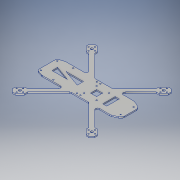
# Autodesk Inventor part: rama
Saved by Autodesk Inventor 2019 (Build 230136000, 136)
## iProperties
Created: 2020-11-11
Part Number: rama
Material: Aluminium 6061
Document SubType Name: Modeling
Designer: Karol
Density: 2.7 g/cm^3
Appearance: Aluminium — płaski
Mass: 121.616 g
Surface Area: 358.369 cm^2
Volume: 45.0429 cm^3
Author: Karol
Autodesk Inventor part; units mm, degrees
ref_plane "YZ Plane" through (0, 0, 0) normal (1, 0, 0) x (0, 1, 0)
ref_plane "XZ Plane" through (0, 0, 0) normal (0, 1, 0) x (-1, 0, 0)
ref_plane "XY Plane" through (0, 0, 0) normal (0, 0, 1) x (1, 0, 0)
sketch "Szkic1" plane through (0, 0, 0) normal (0, 1, 0) x (-1, 0, 0)
  line L0 (-112.8767, 0) -> (86.1409, 0) construction
  circle A0 centre (0, 0) radius 125 construction
  line L1 (0, 0) -> (-129.3005, -129.3005) construction
  line L2 (0, 0) -> (182.8585, 0) construction
  line L3 (0, 0) -> (-129.3005, 129.3005) construction
  circle A1 centre (-88.3883, -88.3883) radius 63.5 construction
  circle A2 centre (-88.3883, 88.3883) radius 63.5 construction
  line L4 (-88.3883, -88.3883) -> (-106.6347, -70.142) construction
  line L5 (-88.3883, -88.3883) -> (-62.5841, -88.3883) construction
  line L6 (0, 0) -> (0, 184.1198) construction
  line L7 (0, 0) -> (129.3005, -129.3005) construction
  line L8 (0, 0) -> (129.3005, 129.3005) construction
  circle A3 centre (88.3883, -88.3883) radius 63.5 construction
  circle A4 centre (88.3883, 88.3883) radius 63.5 construction
  circle A5 centre (70, -24.5) radius 1.5
  circle A6 centre (12, -24.5) radius 1.5
  circle A7 centre (70, 24.5) radius 1.5
  circle A8 centre (12, 24.5) radius 1.5
  line L9 (8.5, -28) -> (100, -28) construction
  line L10 (100, -28) -> (100, 0.6779) construction
  line L11 (8.5, 0) -> (8.5, -28) construction
  circle A9 centre (3.5, -15.283) radius 1.5
  circle A10 centre (-27.066, -15.283) radius 1.5
  circle A11 centre (3.5, 15.283) radius 1.5
  circle A12 centre (-27.066, 15.283) radius 1.5
  line L12 (-19.8579, -29) -> (0.4594, -29)
  line L13 (-75.6604, -82.7315) -> (-23.3934, -30.4645)
  arc A13 (-19.8579, -29) -> (-23.3934, -30.4645) centre (-19.8579, -34) ccw
  line L14 (-19.8579, 29) -> (0.4594, 29)
  arc A14 (-23.3934, 30.4645) -> (-19.8579, 29) centre (-19.8579, 34) ccw
  line L15 (48.1421, -29) -> (92.6893, -29)
  line L16 (19.8579, -29) -> (0.4594, -29)
  arc A15 (23.3934, -30.4645) -> (19.8579, -29) centre (19.8579, -34) ccw
  line L17 (19.8579, 29) -> (0.4594, 29)
  arc A16 (19.8579, 29) -> (23.3934, 30.4645) centre (19.8579, 34) ccw
  line L18 (-88.3883, -88.3883) -> (-88.3883, -65.5663) construction
  circle A17 centre (-80.3883, -88.3883) radius 1.5
  circle A18 centre (-88.3883, -80.3883) radius 1.5
  circle A19 centre (-88.3883, -88.3883) radius 3
  circle A20 centre (-88.3883, -96.3883) radius 1.5
  circle A21 centre (-96.3883, -88.3883) radius 1.5
  line L19 (-82.7315, -75.6604) -> (-89.8026, -75.6604)
  line L20 (-89.8026, -75.6604) -> (-101.1163, -86.9741)
  line L21 (-101.1163, -94.0452) -> (-101.1163, -86.9741)
  line L22 (-101.1163, -94.0452) -> (-97.5807, -97.5807)
  line L23 (-75.6604, -82.7315) -> (-75.6604, -89.8026)
  line L24 (-75.6604, -89.8026) -> (-86.9741, -101.1163)
  line L25 (-94.0452, -101.1163) -> (-86.9741, -101.1163)
  line L26 (-94.0452, -101.1163) -> (-97.5807, -97.5807)
  line L27 (-75.6604, 82.7315) -> (-23.3934, 30.4645)
  circle A22 centre (-80.3883, 88.3883) radius 1.5
  circle A23 centre (-88.3883, 80.3883) radius 1.5
  circle A24 centre (-88.3883, 88.3883) radius 3
  circle A25 centre (-88.3883, 96.3883) radius 1.5
  circle A26 centre (-96.3883, 88.3883) radius 1.5
  line L28 (-82.7315, 75.6604) -> (-89.8026, 75.6604)
  line L29 (-89.8026, 75.6604) -> (-101.1163, 86.9741)
  line L30 (-101.1163, 94.0452) -> (-101.1163, 86.9741)
  line L31 (-101.1163, 94.0452) -> (-97.5807, 97.5807)
  line L32 (-75.6604, 89.8026) -> (-86.9741, 101.1163)
  line L33 (-94.0452, 101.1163) -> (-86.9741, 101.1163)
  line L34 (-94.0452, 101.1163) -> (-97.5807, 97.5807)
  line L35 (-75.6604, 82.7315) -> (-75.6604, 89.8026)
  line L36 (88.3883, -88.3883) -> (106.6347, -70.142) construction
  line L37 (75.6604, -82.7315) -> (23.3934, -30.4645)
  line L38 (88.3883, -88.3883) -> (88.3883, -65.5663) construction
  circle A27 centre (80.3883, -88.3883) radius 1.5
  circle A28 centre (88.3883, -80.3883) radius 1.5
  circle A29 centre (88.3883, -88.3883) radius 3
  circle A30 centre (88.3883, -96.3883) radius 1.5
  circle A31 centre (96.3883, -88.3883) radius 1.5
  line L39 (82.7315, -75.6604) -> (89.8026, -75.6604)
  line L40 (89.8026, -75.6604) -> (101.1163, -86.9741)
  line L41 (101.1163, -94.0452) -> (101.1163, -86.9741)
  line L42 (101.1163, -94.0452) -> (97.5807, -97.5807)
  line L43 (75.6604, -89.8026) -> (86.9741, -101.1163)
  line L44 (94.0452, -101.1163) -> (86.9741, -101.1163)
  line L45 (94.0452, -101.1163) -> (97.5807, -97.5807)
  line L46 (75.6604, -82.7315) -> (75.6604, -89.8026)
  line L47 (75.6604, 82.7315) -> (23.3934, 30.4645)
  line L48 (75.6604, 89.8026) -> (86.9741, 101.1163)
  line L49 (94.0452, 101.1163) -> (86.9741, 101.1163)
  line L50 (82.7315, 75.6604) -> (89.8026, 75.6604)
  circle A32 centre (88.3883, 80.3883) radius 1.5
  circle A33 centre (80.3883, 88.3883) radius 1.5
  circle A34 centre (88.3883, 88.3883) radius 3
  line L51 (89.8026, 75.6604) -> (101.1163, 86.9741)
  circle A35 centre (96.3883, 88.3883) radius 1.5
  line L52 (101.1163, 94.0452) -> (101.1163, 86.9741)
  line L53 (101.1163, 94.0452) -> (97.5807, 97.5807)
  circle A36 centre (88.3883, 96.3883) radius 1.5
  line L54 (94.0452, 101.1163) -> (97.5807, 97.5807)
  line L55 (75.6604, 82.7315) -> (75.6604, 89.8026)
  line L56 (-196.7621, 0) -> (-196.7621, -23) construction
  line L57 (-196.7621, -23) -> (-302.8841, -23) construction
  line L58 (-302.8841, -23) -> (-302.8841, -70.142) construction
  line L59 (-302.8841, -70.142) -> (-413.5658, 0) construction
  line L60 (-196.7621, 0) -> (-196.7621, 23) construction
  line L61 (-196.7621, 23) -> (-302.8841, 23) construction
  line L62 (-302.8841, 23) -> (-302.8841, 70.142) construction
  line L63 (-302.8841, 70.142) -> (-413.5658, 0) construction
  line L64 (-82.7315, -75.6604) -> (-44.6066, -37.5355)
  arc A37 (-44.6066, -37.5355) -> (-48.1421, -29) centre (-48.1421, -34) ccw
  line L65 (82.7315, -75.6604) -> (44.6066, -37.5355)
  arc A38 (48.1421, -29) -> (44.6066, -37.5355) centre (48.1421, -34) ccw
  line L66 (94.2344, -28.7553) -> (106.5451, -24.7553)
  line L67 (110, -20) -> (110, 0)
  arc A39 (92.6893, -29) -> (94.2344, -28.7553) centre (92.6893, -24) ccw
  arc A40 (106.5451, -24.7553) -> (110, -20) centre (105, -20) ccw
  line L68 (-48.1421, -29) -> (-73.1421, -29)
  line L69 (-77.0275, -28.2143) -> (-88.8853, -23.2143)
  line L70 (-95, -14) -> (-95, 0)
  arc A41 (-77.0275, -28.2143) -> (-73.1421, -29) centre (-73.1421, -19) ccw
  arc A42 (-95, -14) -> (-88.8853, -23.2143) centre (-85, -14) ccw
  line L71 (48.1421, 29) -> (92.6893, 29)
  line L72 (-82.7315, 75.6604) -> (-44.6066, 37.5355)
  arc A43 (-48.1421, 29) -> (-44.6066, 37.5355) centre (-48.1421, 34) ccw
  arc A44 (44.6066, 37.5355) -> (48.1421, 29) centre (48.1421, 34) ccw
  line L73 (82.7315, 75.6604) -> (44.6066, 37.5355)
  line L74 (94.2344, 28.7553) -> (106.5451, 24.7553)
  line L75 (110, 20) -> (110, 0)
  arc A45 (110, 20) -> (106.5451, 24.7553) centre (105, 20) ccw
  line L76 (-48.1421, 29) -> (-73.1421, 29)
  line L77 (-77.0275, 28.2143) -> (-88.8853, 23.2143)
  line L78 (-95, 14) -> (-95, 0)
  arc A46 (-73.1421, 29) -> (-77.0275, 28.2143) centre (-73.1421, 19) ccw
  arc A47 (-88.8853, 23.2143) -> (-95, 14) centre (-85, 14) ccw
  arc A48 (94.2344, 28.7553) -> (92.6893, 29) centre (92.6893, 24) ccw
  point P0 (-96.6274, -86.0208)
  point P1 (-104.1875, -93.5809)
  point P2 (-99.7021, -99.7021)
  point P3 (-95, -29)
  point P4 (36.0711, -29)
  point P5 (93.4812, -29)
  point P6 (-85.5599, -88.3883)
  point P7 (-96.6274, 86.0208)
  point P8 (-85.5599, 88.3883)
  point P9 (96.6274, -86.0208)
  point P10 (104.1875, -93.5809)
  point P11 (99.7021, -99.7021)
  point P12 (85.5599, -88.3883)
  point P13 (96.6274, 86.0208)
  point P14 (85.5599, 88.3883)
  dimension "d0" = 250
  dimension "d1" = 135
  dimension "d3" = 127
  dimension "d4" = 127
  dimension "d10" = 135
  dimension "d12" = 3
  dimension "d13" = 24.5
  dimension "d14" = 58
  dimension "d15" = 70
  dimension "d16" = 3.5
  dimension "d17" = 28
  dimension "d19" = 30
  dimension "d20" = 3
  dimension "d22" = 5
  dimension "d23" = 15.283
  dimension "d32" = 5
  dimension "d37" = 30.566
  dimension "d64" = 3
  dimension "d65" = 8
  dimension "d66" = 8
  dimension "d67" = 6
  dimension "d70" = 10
  dimension "d73" = 5
  dimension "d74" = 13
  dimension "d75" = 5
  dimension "d76" = 5
  dimension "d77" = 110
  dimension "d78" = 20
  dimension "d79" = 29
  dimension "d80" = 18
  dimension "d81" = 91.5
  dimension "d82" = 10
  dimension "d83" = 95
  dimension "d84" = 14
  dimension "d85" = 25
  constraints: 158 end point, 103 symmetric about line, 49 centre point, 34 point on circle, 16 point on line, 13 tangent, 7 horizontal, 5 coincident, 5 equal radius, 5 perpendicular, 4 parallel, 4 vertical, 2 equal length, 1 collinear, 33 other
  measures "d0" diameter of A0
  measures "d1" angle of L1 L2
  measures "d3" diameter of A1
  measures "d4" diameter of A2
  measures "d10" angle of L5 L4
  measures "d12" diameter of A5
  measures "d13" vertical distance of point (0, 0) A5.centre
  measures "d14" distance of A5.centre A6.centre
  measures "d15" distance from line of L6 A5.centre
  measures "d16" distance from line of L11 A6.centre
  measures "d17" distance between parallel lines of L0 L9
  measures "d19" distance from line of A5.centre L10
  measures "d20" diameter of A9
  measures "d22" distance from line of A9.centre L11
  measures "d23" distance from line of L0 A9.centre
  measures "d32" radius of A13
  measures "d37" distance of A10.centre A9.centre
  measures "d64" diameter of A17
  measures "d65" distance from line of L5 A18.centre
  measures "d66" distance from line of L18 A17.centre
  measures "d67" diameter of A19
  measures "d70" distance between parallel lines of L1 L20
  measures "d73" distance from line of L1 L19.start
  measures "d74" distance from line of L22 A19.centre
  measures "d75" radius of A37
  measures "d76" radius of A39
  measures "d77" distance between parallel lines of L6 L67
  measures "d78" distance from line of L0 A40.centre
  measures "d79" distance between parallel lines of L0 L15
  measures "d80" angle of L66 L15
  measures "d81" distance between parallel lines of L10 L11
  measures "d82" radius of A41
  measures "d83" distance between parallel lines of L6 L70
  measures "d84" distance from line of L0 A42.centre
  measures "d85" horizontal distance of A37.centre A41.centre
extrude "Wyciągnięcie proste5" add sketch "Szkic1" along normal blind 3
sketch "Szkic2" plane through (0, 3, 0) normal (0, 1, 0) x (1, 0, 0)
  circle A0 centre (-88.3883, 88.3883) radius 3 projected
  circle A1 centre (-88.3883, -88.3883) radius 3 projected
  circle A2 centre (88.3883, -88.3883) radius 3 projected
  circle A3 centre (88.3883, 88.3883) radius 3 projected
  circle A4 centre (-88.3883, 96.3883) radius 1.5 projected
  circle A5 centre (-96.3883, 88.3883) radius 1.5 projected
  circle A6 centre (-88.3883, 80.3883) radius 1.5 projected
  circle A7 centre (-80.3883, 88.3883) radius 1.5 projected
  circle A8 centre (-96.3883, -88.3883) radius 1.5 projected
  circle A9 centre (-88.3883, -96.3883) radius 1.5 projected
  circle A10 centre (-88.3883, -80.3883) radius 1.5 projected
  circle A11 centre (-80.3883, -88.3883) radius 1.5 projected
  circle A12 centre (88.3883, -96.3883) radius 1.5 projected
  circle A13 centre (96.3883, -88.3883) radius 1.5 projected
  circle A14 centre (80.3883, -88.3883) radius 1.5 projected
  circle A15 centre (88.3883, -80.3883) radius 1.5 projected
  circle A16 centre (96.3883, 88.3883) radius 1.5 projected
  circle A17 centre (88.3883, 96.3883) radius 1.5 projected
  circle A18 centre (88.3883, 80.3883) radius 1.5 projected
  circle A19 centre (80.3883, 88.3883) radius 1.5 projected
  circle A20 centre (-3.5, -15.283) radius 1.5 projected
  circle A21 centre (27.066, -15.283) radius 1.5 projected
  circle A22 centre (27.066, 15.283) radius 1.5 projected
  circle A23 centre (-3.5, 15.283) radius 1.5 projected
  circle A24 centre (-70, -24.5) radius 1.5 projected
  circle A25 centre (-12, -24.5) radius 1.5 projected
  circle A26 centre (-12, 24.5) radius 1.5 projected
  circle A27 centre (-70, 24.5) radius 1.5 projected
  line L0 (82.7315, 75.6604) -> (89.8026, 75.6604) projected
  line L1 (89.8026, 75.6604) -> (101.1163, 86.9741) projected
  line L2 (101.1163, 86.9741) -> (101.1163, 94.0452) projected
  line L3 (101.1163, 94.0452) -> (94.0452, 101.1163) projected
  line L4 (94.0452, 101.1163) -> (86.9741, 101.1163) projected
  line L5 (86.9741, 101.1163) -> (75.6604, 89.8026) projected
  line L6 (75.6604, 89.8026) -> (75.6604, 82.7315) projected
  line L7 (75.6604, 82.7315) -> (23.3934, 30.4645) projected
  arc A28 (19.8579, 29) -> (23.3934, 30.4645) centre (19.8579, 34) ccw projected
  line L8 (19.8579, 29) -> (-19.8579, 29) projected
  arc A29 (-23.3934, 30.4645) -> (-19.8579, 29) centre (-19.8579, 34) ccw projected
  line L9 (-23.3934, 30.4645) -> (-75.6604, 82.7315) projected
  line L10 (-75.6604, 82.7315) -> (-75.6604, 89.8026) projected
  line L11 (-75.6604, 89.8026) -> (-86.9741, 101.1163) projected
  line L12 (-86.9741, 101.1163) -> (-94.0452, 101.1163) projected
  line L13 (-94.0452, 101.1163) -> (-101.1163, 94.0452) projected
  line L14 (-101.1163, 94.0452) -> (-101.1163, 86.9741) projected
  line L15 (-101.1163, 86.9741) -> (-89.8026, 75.6604) projected
  line L16 (-89.8026, 75.6604) -> (-82.7315, 75.6604) projected
  line L17 (-82.7315, 75.6604) -> (-44.6066, 37.5355) projected
  arc A30 (-48.1421, 29) -> (-44.6066, 37.5355) centre (-48.1421, 34) ccw projected
  line L18 (-48.1421, 29) -> (-92.6893, 29) projected
  arc A31 (-92.6893, 29) -> (-94.2344, 28.7553) centre (-92.6893, 24) ccw projected
  line L19 (-94.2344, 28.7553) -> (-106.5451, 24.7553) projected
  arc A32 (-106.5451, 24.7553) -> (-110, 20) centre (-105, 20) ccw projected
  line L20 (-110, 20) -> (-110, -20) projected
  arc A33 (-110, -20) -> (-106.5451, -24.7553) centre (-105, -20) ccw projected
  line L21 (-106.5451, -24.7553) -> (-94.2344, -28.7553) projected
  arc A34 (-94.2344, -28.7553) -> (-92.6893, -29) centre (-92.6893, -24) ccw projected
  line L22 (-92.6893, -29) -> (-48.1421, -29) projected
  arc A35 (-44.6066, -37.5355) -> (-48.1421, -29) centre (-48.1421, -34) ccw projected
  line L23 (-44.6066, -37.5355) -> (-82.7315, -75.6604) projected
  line L24 (-82.7315, -75.6604) -> (-89.8026, -75.6604) projected
  line L25 (-89.8026, -75.6604) -> (-101.1163, -86.9741) projected
  line L26 (-101.1163, -86.9741) -> (-101.1163, -94.0452) projected
  line L27 (-101.1163, -94.0452) -> (-94.0452, -101.1163) projected
  line L28 (-94.0452, -101.1163) -> (-86.9741, -101.1163) projected
  line L29 (-86.9741, -101.1163) -> (-75.6604, -89.8026) projected
  line L30 (-75.6604, -89.8026) -> (-75.6604, -82.7315) projected
  line L31 (-75.6604, -82.7315) -> (-23.3934, -30.4645) projected
  arc A36 (-19.8579, -29) -> (-23.3934, -30.4645) centre (-19.8579, -34) ccw projected
  line L32 (-19.8579, -29) -> (19.8579, -29) projected
  arc A37 (23.3934, -30.4645) -> (19.8579, -29) centre (19.8579, -34) ccw projected
  line L33 (23.3934, -30.4645) -> (75.6604, -82.7315) projected
  line L34 (75.6604, -82.7315) -> (75.6604, -89.8026) projected
  line L35 (75.6604, -89.8026) -> (86.9741, -101.1163) projected
  line L36 (86.9741, -101.1163) -> (94.0452, -101.1163) projected
  line L37 (94.0452, -101.1163) -> (101.1163, -94.0452) projected
  line L38 (101.1163, -94.0452) -> (101.1163, -86.9741) projected
  line L39 (101.1163, -86.9741) -> (89.8026, -75.6604) projected
  line L40 (89.8026, -75.6604) -> (82.7315, -75.6604) projected
  line L41 (82.7315, -75.6604) -> (44.6066, -37.5355) projected
  arc A38 (48.1421, -29) -> (44.6066, -37.5355) centre (48.1421, -34) ccw projected
  line L42 (48.1421, -29) -> (73.1421, -29) projected
  arc A39 (73.1421, -29) -> (77.0275, -28.2143) centre (73.1421, -19) ccw projected
  line L43 (77.0275, -28.2143) -> (88.8853, -23.2143) projected
  arc A40 (88.8853, -23.2143) -> (95, -14) centre (85, -14) ccw projected
  line L44 (95, -14) -> (95, 14) projected
  arc A41 (95, 14) -> (88.8853, 23.2143) centre (85, 14) ccw projected
  line L45 (88.8853, 23.2143) -> (77.0275, 28.2143) projected
  arc A42 (77.0275, 28.2143) -> (73.1421, 29) centre (73.1421, 19) ccw projected
  line L46 (73.1421, 29) -> (48.1421, 29) projected
  arc A43 (44.6066, 37.5355) -> (48.1421, 29) centre (48.1421, 34) ccw projected
  line L47 (44.6066, 37.5355) -> (82.7315, 75.6604) projected
  circle A44 centre (-3.5, 24.5) radius 1.5
  circle A45 centre (87, 16) radius 1.5
  circle A46 centre (-105, 20) radius 1.5
  line L48 (0, 0) -> (95, 0) construction
  line L49 (0, 0) -> (0, 60.6938) construction
  circle A47 centre (-3.5, -24.5) radius 1.5
  circle A48 centre (87, -16) radius 1.5
  circle A49 centre (-105, -20) radius 1.5
  line L50 (4.283, -7.5) -> (19.283, -7.5)
  line L51 (19.283, -7.5) -> (19.283, 7.5)
  line L52 (19.283, 7.5) -> (4.283, 7.5)
  line L53 (4.283, 7.5) -> (4.283, -7.5)
  line L54 (4.283, -7.5) -> (19.283, 7.5) construction
  line L55 (19.283, -7.5) -> (4.283, 7.5) construction
  line L56 (-95, 12.5) -> (-25, 12.5) construction
  line L57 (-25, 12.5) -> (-25, -12.5) construction
  line L58 (-25, -12.5) -> (-95, -12.5) construction
  line L59 (-95, -12.5) -> (-95, 12.5) construction
  line L60 (-95, 12.5) -> (-25, -12.5) construction
  line L61 (-25, 12.5) -> (-95, -12.5) construction
  line L62 (-3.5, -15.283) -> (-3.5, -8.7545) construction
  line L63 (27.066, -15.283) -> (27.066, -7.574) construction
  line L64 (11.783, 0) -> (11.783, 6.8705) construction
  line L65 (-29, -6.824) -> (-29, 8.5)
  line L66 (-29, 8.5) -> (-71.9071, 8.5)
  line L67 (-71.9071, 8.5) -> (-29, -6.824)
  line L68 (-91, 6.824) -> (-52.7857, -6.824)
  line L69 (-52.7857, -6.824) -> (-91, -6.824)
  line L70 (-91, -6.824) -> (-91, 6.824)
  line L71 (52.066, -15.283) -> (42.066, -15.283)
  line L72 (42.066, -15.283) -> (42.066, 15.283)
  line L73 (42.066, 15.283) -> (52.066, 15.283)
  line L74 (52.066, 15.283) -> (52.066, -15.283)
  line L75 (52.066, -15.283) -> (42.066, 15.283) construction
  line L76 (42.066, -15.283) -> (52.066, 15.283) construction
  point P0 (-60, 0)
  point P1 (-60, 0)
  point P2 (47.066, 0)
  point P3 (47.066, 15.283)
  dimension "d87" = 3
  dimension "d88" = 20
  dimension "d89" = 16
  dimension "d90" = 8
  dimension "d91" = 15
  dimension "d92" = 15
  dimension "d93" = 70
  dimension "d94" = 25
  dimension "d95" = 60
  dimension "d96" = 4
  dimension "d97" = 4
  dimension "d98" = 4
  dimension "d101" = 10
  dimension "d102" = 20
  constraints: 58 end point, 9 midpoint, 7 parallel, 6 centre point, 5 perpendicular, 4 horizontal, 4 horizontal alignment, 4 vertical, 3 symmetric about line, 2 equal radius, 2 point on line, 1 coincident, 1 vertical alignment, 6 other
  measures "d87" diameter of A45
  measures "d88" distance from line of L48 A46.centre
  measures "d89" distance from line of A45.centre L48
  measures "d90" distance from line of L44 A45.centre
  measures "d91" distance of L50.end L51.end
  measures "d92" distance of L51.end L52.end
  measures "d93" distance of L56.start L56.end
  measures "d94" distance of L56.end L57.end
  measures "d95" distance of point (-60, 0) L48.start
  measures "d96" distance between parallel lines of L60 L67
  measures "d97" distance between parallel lines of L60 L68
  measures "d98" distance between parallel lines of L59 L70
  measures "d101" distance of L72.end L73.end
  measures "d102" horizontal distance of L63.start point (47.066, 0)
extrude "Wyciągnięcie proste6" cut sketch "Szkic2" against normal through all contours A44 | A45 | A46 | A47 | A48 | A49 | L53 L52 L51 L50 | L67 L66 L65 | L68 L69 L70 | L71 L72 L73 L74
